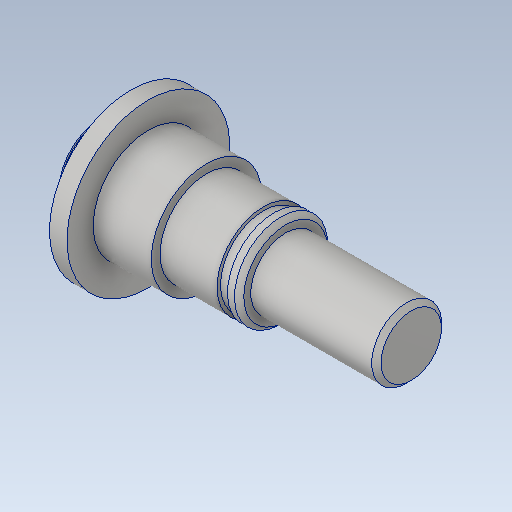
# Autodesk Inventor part: UpperLowerArm_JointShaft
Saved by Autodesk Inventor 2021.4 (Build 254397000, 397)
## iProperties
Created: 2022-07-06
Part Number: UpperLowerArm_JointShaft
Material: Aluminum 6061
Document SubType Name: Modeling
Designer: alexw
Density: 2.7 g/cm^3
Appearance: Aluminum - Flat
Mass: 3.5038 g
Surface Area: 10.1872 cm^2
Volume: 1.2977 cm^3
ShaftFixation_UpperLower_Height: 8,000 mm
Bearing_OuterRing_Dia: 10,500 mm
MountingPlate_MEnc_Distance: 14,100 mm
Cover_MountingPlate_Thickness: 1,500 mm
Author: alexw
Autodesk Inventor part; units mm, degrees
ref_plane "YZ Plane" through (0, 0, 0) normal (1, 0, 0) x (0, 1, 0)
ref_plane "XZ Plane" through (0, 0, 0) normal (0, 1, 0) x (-1, 0, 0)
sketch "Sketch1" plane through (0, 0, 0) normal (0, 0, 1) x (1, 0, 0)
  line L0 (15.9, 4) -> (15.9, 3)
  line L1 (15.9, 3) -> (26.7, 3)
  line L2 (26.7, 3) -> (26.7, 0)
  line L3 (26.7, 0) -> (0, 0)
  line L4 (0, 0) -> (0, 4)
  line L5 (4.1, 4.75) -> (9.1, 4.75)
  line L6 (9.1, 4.75) -> (9.1, 4)
  line L7 (0, 4) -> (2.6, 4)
  line L8 (14, 4) -> (14, 3.7)
  line L9 (14, 3.7) -> (14.9, 3.7)
  line L10 (14.9, 3.7) -> (14.9, 4)
  line L11 (9.1, 4) -> (14, 4)
  line L12 (14.9, 4) -> (15.9, 4)
  line L13 (14.1, 4) -> (14.1, 0) construction
  line L14 (4.1, 4.75) -> (4.1, 0) construction
  line L15 (16.7, 3) -> (16.7, 0) construction
  line L16 (18.2, 3) -> (18.2, 0) construction
  line L17 (2.6, 4) -> (2.6, 7)
  line L18 (2.6, 7) -> (4.1, 7)
  line L19 (4.1, 7) -> (4.1, 4.75)
  line L20 (9.1, 4) -> (9.1, 0) construction
  line L21 (6.1, 4.75) -> (6.1, 0) construction
  dimension "d0" = 6
  dimension "d2" = 9.5
  dimension "d3" = 8
  dimension "d7" = 0.9
  dimension "d8" = 7.4
  dimension "d9" = 1
  dimension "Cover_MountingPlate_Thickness" = 1.5
  dimension "d23" = 0.8
  dimension "MountingPlate_MEnc_Distance" = 14.1
  dimension "d25" = 8.5
  dimension "d29" = 14
  dimension "d31" = 1.5
  dimension "d32" = 2.6
  dimension "d33" = 0.1
  dimension "d34" = 5
  dimension "d35" = 8
  dimension "d36" = 2
  constraints: 44 end point, 21 perpendicular, 11 point on line, 5 horizontal, 3 collinear, 1 vertical
  measures "d0" diameter of L1 L3
  measures "d2" diameter of L5 L3
  measures "d3" diameter of L7 L3
  measures "d7" distance between parallel lines of L10 L8
  measures "d8" diameter of L9 L3
  measures "d9" distance between parallel lines of L0 L10
  measures "Cover_MountingPlate_Thickness" distance between parallel lines of L16 L15
  measures "d23" distance from line of L0.end L15
  measures "MountingPlate_MEnc_Distance" distance between parallel lines of L16 L14
  measures "d25" distance between parallel lines of L2 L16
  measures "d29" diameter of L18 L3
  measures "d31" distance between parallel lines of L19 L17
  measures "d32" distance between parallel lines of L4 L17
  measures "d33" distance between parallel lines of L8 L13
  measures "d34" distance between parallel lines of L20 L13
  measures "d35" distance between parallel lines of L21 L13
  measures "d36" distance between parallel lines of L14 L21
revolve "Revolution1" add sketch "Sketch1" angle 360 about axis through (26.7, 0, 0) along (-1, 0, 0)
chamfer "Chamfer1" distance 0.4 angle 45 3 edges at (0, -4, 0) (26.7, -3, 0) (15.9, -4, 0)
ref_plane "Work Plane4" through (26.7, 0, 0) normal (1, 0, 0) x (0, 0, -1)
ref_plane "Work Plane3" through (18.2, 0, 0) normal (1, 0, 0) x (0, 0, -1)
sketch "Sketch2" plane through (0, 0, 0) normal (-1, 0, 0) x (0, 0, 1)
  point P0 (0, 0)
  point P1 (0, 0)
  constraints: 1 coincident
hole "Hole1" at (0, 0, 0) direction (1, 0, 0) diameter 3.242 depth 6 tip angle 118 thread size "M4x0.7" class "6H" standard "ISO Metric profile"
chamfer "Chamfer2" distance 0.5 angle 45 1 edges at (0, 0, -1.621)
ref_plane "Work Plane2" through (16.7, 0, 0) normal (1, 0, 0) x (0, 0, -1)
equation "\"d35\" = ShaftFixation_UpperLower_Height"
equation "\"d36\" = BasePlate_UpperLowerConnector_Height"
equation "\"d18\" = d23"
equation "\"d19\" = Cover_MountingPlate_Thickness"
equation "\"d20\" = d25"
equation "\"ShaftFixation_UpperLower_Height\" = 8"
equation "\"BasePlate_UpperLowerConnector_Height\" = 2"
body "Solid1"
